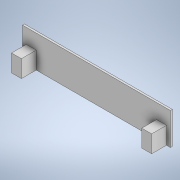
# Autodesk Inventor part: pièce_chassis
Saved by Autodesk Inventor 2020.2 (Build 242310000, 310)
## iProperties
Created: 2020-02-25
Part Number: pièce_chassis
Material: Générique
Document SubType Name: Modeling
Designer: anton
Density: 1 g/cm^3
Appearance: Par défaut
Author: anton
Autodesk Inventor part; units mm, degrees
ref_plane "YZ Plane" through (0, 0, 0) normal (1, 0, 0) x (0, 1, 0)
ref_plane "XZ Plane" through (0, 0, 0) normal (0, 1, 0) x (-1, 0, 0)
ref_plane "XY Plane" through (0, 0, 0) normal (0, 0, 1) x (1, 0, 0)
sketch "Esquisse1" plane through (0, 0, 0) normal (0, 0, 1) x (1, 0, 0)
  line L0 (-141.642, 40.418) -> (158.358, 40.418)
  line L1 (158.358, 40.418) -> (158.358, -24.582)
  line L2 (158.358, -24.582) -> (-141.642, -24.582)
  line L3 (-141.642, -24.582) -> (-141.642, 40.418)
  point P0 (0, 0)
  dimension "d0" = 300
  dimension "d1" = 65
  constraints: 8 end point, 2 parallel, 1 horizontal, 1 perpendicular
  measures "d0" distance of L0.start L0.end
  measures "d1" distance of L2.end L0.start
extrude "Extrusion1" add sketch "Esquisse1" along normal blind 4
sketch "Esquisse2" plane through (0, 0, 4) normal (0, 0, 1) x (1, 0, 0)
  line L0 (-133.642, 10.418) -> (-113.642, 10.418)
  line L1 (-113.642, 10.418) -> (-113.642, -24.582)
  line L2 (-113.642, -24.582) -> (-133.642, -24.582)
  line L3 (-133.642, -24.582) -> (-133.642, 10.418)
  line L4 (130.358, 10.418) -> (150.358, 10.418)
  line L5 (150.358, 10.418) -> (150.358, -24.582)
  line L6 (150.358, -24.582) -> (130.358, -24.582)
  line L7 (130.358, -24.582) -> (130.358, 10.418)
  line L8 (-141.642, -24.582) -> (158.358, -24.582) projected
  line L9 (-141.642, 40.418) -> (-141.642, -24.582) projected
  line L10 (158.358, -24.582) -> (158.358, 40.418) projected
  point P0 (0, 0)
  dimension "d4" = 0
  dimension "d5" = 0
  dimension "d6" = 35
  dimension "d7" = 35
  dimension "d8" = 20
  dimension "d9" = 20
  dimension "d10" = 8
  dimension "d11" = 8
  constraints: 16 end point, 4 parallel, 2 horizontal, 2 perpendicular
  measures "d4" distance between parallel lines of L8 L2
  measures "d5" distance between parallel lines of L8 L6
  measures "d6" distance of L4.end L5.end
  measures "d7" distance of L2.end L0.start
  measures "d8" distance of L0.start L0.end
  measures "d9" distance of L4.start L4.end
  measures "d10" distance between parallel lines of L9 L3
  measures "d11" distance between parallel lines of L10 L5
extrude "Extrusion2" add sketch "Esquisse2" along normal blind 30
sketch "Esquisse3" plane through (0, 0, 0) normal (0, 0, -1) x (-1, 0, 0)
  line L0 (-148.358, 35.418) -> (131.642, 35.418)
  line L1 (131.642, 35.418) -> (131.642, 25.418)
  line L2 (131.642, 25.418) -> (-148.358, 25.418)
  line L3 (-148.358, 25.418) -> (-148.358, 35.418)
  line L4 (-148.358, 20.418) -> (131.642, 20.418)
  line L5 (131.642, 20.418) -> (131.642, 10.418)
  line L6 (131.642, 10.418) -> (-148.358, 10.418)
  line L7 (-148.358, 10.418) -> (-148.358, 20.418)
  line L8 (-158.358, 40.418) -> (141.642, 40.418) projected
  line L9 (-148.358, 5.418) -> (131.642, 5.418)
  line L10 (131.642, 5.418) -> (131.642, -4.582)
  line L11 (131.642, -4.582) -> (-148.358, -4.582)
  line L12 (-148.358, -4.582) -> (-148.358, 5.418)
  line L13 (-148.358, -9.582) -> (131.642, -9.582)
  line L14 (131.642, -9.582) -> (131.642, -19.582)
  line L15 (131.642, -19.582) -> (-148.358, -19.582)
  line L16 (-148.358, -19.582) -> (-148.358, -9.582)
  line L17 (141.642, -24.582) -> (-158.358, -24.582) projected
  line L18 (-158.358, -24.582) -> (-158.358, 40.418) projected
  dimension "d14" = 5
  dimension "d15" = 10
  dimension "d16" = 5
  dimension "d17" = 10
  dimension "d20" = 5
  dimension "d21" = 10
  dimension "d22" = 5
  dimension "d23" = 10
  dimension "d24" = 280
  dimension "d25" = 280
  dimension "d26" = 280
  dimension "d27" = 280
  dimension "d28" = 10
  dimension "d29" = 10
  dimension "d30" = 10
  dimension "d31" = 10
  constraints: 32 end point, 8 parallel, 4 horizontal, 4 perpendicular, 1 point on line
  measures "d14" distance between parallel lines of L8 L0
  measures "d15" distance of L2.end L0.start
  measures "d16" distance between parallel lines of L4 L2
  measures "d17" distance of L6.end L4.start
  measures "d20" distance between parallel lines of L17 L15
  measures "d21" distance of L15.end L13.start
  measures "d22" distance between parallel lines of L13 L11
  measures "d23" distance of L11.end L9.start
  measures "d24" distance of L0.start L0.end
  measures "d25" distance of L4.start L4.end
  measures "d26" distance of L9.start L9.end
  measures "d27" distance of L14.end L15.end
  measures "d28" distance between parallel lines of L18 L16
  measures "d29" distance between parallel lines of L18 L12
  measures "d30" distance between parallel lines of L18 L7
  measures "d31" distance between parallel lines of L18 L3
extrude "Extrusion3" cut sketch "Esquisse3" against normal blind 1
